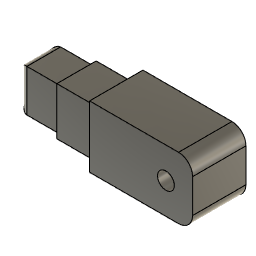
Motor v1 (Autodesk Fusion 360 design; units mm, degrees)
Autodesk Fusion 360 part; units mm, degrees
sketch "Sketch1" plane through (0, 0, 0) normal (0, 0, 1) x (1, 0, 0) in component "Motor"
  line L0 (32.5, 9.5) -> (-32.5, 9.5)
  line L1 (-32.5, 9.5) -> (-32.5, -9.5)
  line L2 (-32.5, -9.5) -> (32.5, -9.5)
  line L3 (32.5, -9.5) -> (32.5, 9.5)
  line L4 (32.5, 9.5) -> (-32.5, -9.5) construction
  line L5 (-32.5, 9.5) -> (32.5, -9.5) construction
  dimension "d1" = 65
  dimension "d2" = 19
  constraint horizontal L0
  constraint perpendicular L0 L1
  constraint parallel L0 L2
  constraint parallel L1 L3
  constraint coincident L4 origin
  constraint coincident L5 origin
  measures "d1" distance of L1.end L2.end
  measures "d2" distance of L0.end L1.end
extrude "Extrude1" add sketch "Sketch1" along normal blind 25 in component "Motor"
extrude "Extrude2" cut 1 faces at (-10.8333, -3.1667, 25) along direction (0, 0, -1) blind 3 in component "Motor"
extrude "Extrude3" cut 1 faces at (-32.5, 3.1667, 14.6667) along direction (1, 0, 0) blind 28.3 in component "Motor"
sketch "Sketch2" plane through (-4.2, 0, 0) normal (-1, 0, 0) x (0, -1, 0) in component "Motor"
  line L0 (9.5, 22) -> (-9.5, 22)
  line L1 (-9.5, 22) -> (-9.5, 0)
  line L2 (-9.5, 0) -> (9.5, 0)
  line L3 (9.5, 0) -> (9.5, 22)
  line L4 (-9.5, 22) -> (9.5, 22)
  line L5 (9.5, 22) -> (9.5, 0)
  line L6 (9.5, 0) -> (-9.5, 0)
  line L7 (-9.5, 0) -> (-9.5, 22)
  line L8 (-7, 19) -> (7, 19)
  line L9 (7, 19) -> (7, 2)
  line L10 (7, 2) -> (-7, 2)
  line L11 (-7, 2) -> (-7, 19)
  line L12 (-6, 18) -> (6, 18)
  line L13 (6, 18) -> (6, 3)
  line L14 (6, 3) -> (-6, 3)
  line L15 (-6, 3) -> (-6, 18)
  constraint horizontal L4
  constraint vertical L5
  constraint horizontal L6
  constraint vertical L7
  constraint coincident L2.end L3.start
  constraint coincident L0.end L1.start
  constraint horizontal L8
  constraint vertical L9
  constraint horizontal L10
  constraint vertical L11
  constraint horizontal L12
  constraint vertical L13
  constraint horizontal L14
  constraint vertical L15
extrude "Extrude4" add sketch "Sketch2" along normal blind 28.3 contours L8 L9 L10 L11 | L12 L13 L14 L15 in component "Motor"
fillet "Fillet1" radius 5 2 edges at (32.5, 0, 22) (32.5, 0, 0) in component "Motor"
extrude "Extrude5" cut 1 faces at (-32.5, 2.3333, 7.6667) along direction (1, 0, 0) blind 14.15 in component "Motor"
extrude "Extrude6" add sketch "Sketch2" along normal blind 28.3 contours L12 L13 L14 L15 in component "Motor"
fillet "Fillet2" radius 2.5 1 faces at (-32.5, 2, 13) in component "Motor"
sketch "Sketch3" plane through (0, -9.5, 0) normal (0, -1, 0) x (1, 0, 0) in component "Motor"
  arc A0 (27.5, 0) -> (32.5, 5) centre (27.5, 5) ccw
  line L0 (32.5, 5) -> (32.5, 17)
  arc A1 (32.5, 17) -> (27.5, 22) centre (27.5, 17) ccw
  line L1 (27.5, 22) -> (-4.2, 22)
  line L2 (-4.2, 22) -> (-4.2, 0)
  line L3 (-4.2, 0) -> (27.5, 0)
  line L4 (-4.2, 22) -> (27.6, 22)
  line L5 (32.6, 17) -> (32.6, 5)
  line L6 (27.6, 0) -> (-4.2, 0)
  line L7 (-4.2, 0) -> (-4.2, 22)
  arc A2 (32.6, 17) -> (27.6, 22) centre (27.6, 17) ccw
  arc A3 (27.6, 0) -> (32.6, 5) centre (27.6, 5) ccw
  circle A4 centre (23, 11) radius 3
  point P0 (32.6, 22)
  dimension "d19" = 36.8
  dimension "d20" = 5
  dimension "d21" = 6
  constraint horizontal L4
  constraint vertical L5
  constraint horizontal L6
  constraint vertical L7
  constraint coincident L1.end L2.start
  constraint coincident P0 L4
  constraint coincident P0 L5
  constraint tangent L4 A2
  constraint tangent L5 A2
  constraint tangent L5 A3
  constraint tangent L6 A3
  constraint equal A2 A3
  measures "d19" distance of L1.end P0
  measures "d20" radius of A2
  measures "d21" diameter of A4
extrude "Extrude7" cut sketch "Sketch3" against normal blind 56 contours A4 in component "Motor"
component "Motor" placed x (1, 0, 0) y (0, 1, 0) z (0, 0, 1) at (0, 0, 0)
equation "d13 = ( -28.3 / 2 ) * 1 mm"
